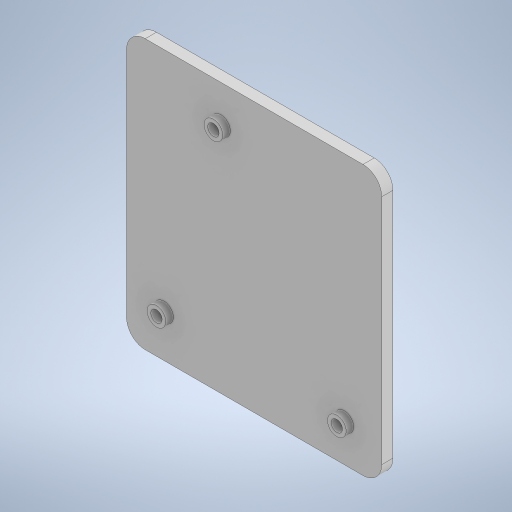
# Autodesk Inventor part: ArduSimple BasePlate FlatAdapter
Saved by Autodesk Inventor 2023 (Build 270158000, 158)
## iProperties
Created: 2023-01-11
Part Number: ArduSimple BasePlate FlatAdapter
Material: Generic
Document SubType Name: Modeling
Designer: Administrator
Density: 1 g/cm^3
Appearance: Default
Author: Administrator
Autodesk Inventor part; units mm, degrees
ref_plane "YZ Plane" through (0, 0, 0) normal (1, 0, 0) x (0, 1, 0)
ref_plane "XZ Plane" through (0, 0, 0) normal (0, 1, 0) x (-1, 0, 0)
ref_plane "XY Plane" through (0, 0, 0) normal (0, 0, 1) x (1, 0, 0)
sketch "Sketch1" plane through (0, 0, 0) normal (0, 0, 1) x (1, 0, 0)
  circle A0 centre (-48.26, 7.249) radius 1.5
  circle A1 centre (0, 5.979) radius 1.5
  circle A2 centre (-33.02, 58.049) radius 1.5
  line L0 (-53.26, 68.049) -> (5, 68.049)
  line L1 (10, 63.049) -> (10, 0.979)
  line L2 (5, -4.021) -> (-53.26, -4.021)
  line L3 (-58.26, 0.979) -> (-58.26, 63.049)
  arc A3 (-53.26, 68.049) -> (-58.26, 63.049) centre (-53.26, 63.049) ccw
  arc A4 (10, 63.049) -> (5, 68.049) centre (5, 63.049) ccw
  arc A5 (5, -4.021) -> (10, 0.979) centre (5, 0.979) ccw
  arc A6 (-58.26, 0.979) -> (-53.26, -4.021) centre (-53.26, 0.979) ccw
  point P0 (0, 0)
  point P1 (-28.5358, 0.3645)
  point P2 (-23.2442, 0.3645)
  dimension "d1" = 3
  dimension "d2" = 3
  dimension "d3" = 48.26
  dimension "d5" = 1.27
  dimension "d6" = 3
  dimension "d8" = 15.24
  dimension "d9" = 50.8
  dimension "d10" = 10
  dimension "d12" = 10
  dimension "d13" = 10
  dimension "d14" = 10
  dimension "d15" = 5
  constraints: 8 end point, 8 point on circle, 8 tangent, 7 centre point, 3 equal radius, 2 parallel, 1 horizontal, 1 perpendicular
  measures "d1" diameter of A0
  measures "d2" diameter of A1
  measures "d3" horizontal distance of A1.centre A0.centre
  measures "d5" vertical distance of A1.centre A0.centre
  measures "d6" diameter of A2
  measures "d8" horizontal distance of A0.centre A2.centre
  measures "d9" vertical distance of A2.centre A0.centre
  measures "d10" distance from line of L1 point (0, 0)
  measures "d12" distance from line of A2.centre L0
  measures "d13" distance from line of L2 A1.centre
  measures "d14" distance from line of A0.centre L3
  measures "d15" radius of A3
extrude "Extrusion1" add sketch "Sketch1" along normal blind 3
sketch "Sketch2" plane through (0, 0, 3) normal (0, 0, 1) x (1, 0, 0)
  circle A0 centre (-33.02, 58.049) radius 1.5 projected
  circle A1 centre (-33.02, 58.049) radius 2.5
  circle A2 centre (0, 5.979) radius 1.5 projected
  circle A3 centre (0, 5.979) radius 2.5
  circle A4 centre (-48.26, 7.249) radius 1.5 projected
  circle A5 centre (-48.26, 7.249) radius 2.5
  circle A6 centre (-33.02, 58.049) radius 1.5
  circle A7 centre (-48.26, 7.249) radius 1.5
  circle A8 centre (0, 5.979) radius 1.5
  point P0 (0, 0)
  dimension "d18" = 5
  dimension "d19" = 5
  dimension "d20" = 5
  constraints: 6 centre point, 6 coincident, 3 concentric
  measures "d18" diameter of A1
  measures "d19" diameter of A3
  measures "d20" diameter of A5
extrude "Extrusion2" add sketch "Sketch2" along normal blind 2
body "Solid1"
